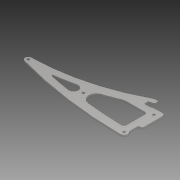
# Autodesk Inventor part: Накладка_4.1.4_3.1_захват(10мм)
Saved by Autodesk Inventor 2016 (Build 200138000, 138)
## iProperties
Created: 2020-03-12
Part Number: Накладка_4.1.4_3.1_захват(10мм)
Material: Поликарбонат, прозрачный
Document SubType Name: Modeling
Designer: Рябов
Density: 1.2 g/cm^3
Appearance: Поликарбонат — прозрачный
Mass: 7.31386 g
Surface Area: 73.6332 cm^2
Volume: 6.09488 cm^3
Author: Рябов
Autodesk Inventor part; units mm, degrees
ref_plane "YZ Plane" through (0, 0, 0) normal (1, 0, 0) x (0, 1, 0)
ref_plane "XZ Plane" through (0, 0, 0) normal (0, 1, 0) x (-1, 0, 0)
ref_plane "XY Plane" through (0, 0, 0) normal (0, 0, 1) x (1, 0, 0)
sketch "Эскиз1" plane through (0, 0, 0) normal (0, 0, 1) x (1, 0, 0)
  circle A0 centre (6.4823, -1.4624) radius 1.65
  circle A1 centre (6.4823, -40.9716) radius 1.65 construction
  arc A2 (-57.7734, 9.189) -> (-62.7021, 3.6942) centre (-59.7433, 5.998) ccw construction
  circle A3 centre (-59.7433, 5.998) radius 1.65 construction
  line L0 (-4.1893, 7.0157) -> (-4.1893, 7.0357) construction
  line L1 (-4.1893, 7.0357) -> (-3.1893, 7.0357) construction
  line L2 (-3.1893, 7.0357) -> (-3.1893, 7.0157) construction
  line L3 (-3.1893, 7.0157) -> (-1.1893, 7.0157) construction
  line L4 (-1.1893, 7.0157) -> (-1.1893, 7.0357) construction
  line L5 (-1.1893, 7.0357) -> (0.8107, 7.0357) construction
  line L6 (0.8107, 7.0357) -> (0.8107, 6.6351) construction
  line L7 (0.8107, 6.6351) -> (-1.1893, 6.6351) construction
  line L8 (-1.1893, 6.6351) -> (-1.1893, 6.6551) construction
  line L9 (-1.1893, 6.6551) -> (-3.1893, 6.6551) construction
  line L10 (-3.1893, 6.6551) -> (-3.1893, 6.6351) construction
  line L11 (-3.1893, 6.6351) -> (-4.1893, 6.6351) construction
  line L12 (-4.1893, 6.6351) -> (-4.1893, 6.6551) construction
  line L13 (-4.1893, 6.6551) -> (-6.1893, 6.6551) construction
  line L14 (-6.1893, 6.6551) -> (-6.1893, 6.6351) construction
  line L15 (-6.1893, 6.6351) -> (-7.1893, 6.6351) construction
  line L16 (-7.1893, 6.6351) -> (-7.1893, 6.6551) construction
  line L17 (-7.1893, 6.6551) -> (-9.1893, 6.6551) construction
  line L18 (-9.1893, 6.6551) -> (-9.1893, 6.6351) construction
  line L19 (-9.1893, 6.6351) -> (-11.1893, 6.6351) construction
  line L20 (-11.1893, 6.6351) -> (-11.1893, 7.0357) construction
  line L21 (-11.1893, 7.0357) -> (-9.1893, 7.0357) construction
  line L22 (-9.1893, 7.0357) -> (-9.1893, 7.0157) construction
  line L23 (-9.1893, 7.0157) -> (-7.1893, 7.0157) construction
  line L24 (-7.1893, 7.0157) -> (-7.1893, 7.0357) construction
  line L25 (-7.1893, 7.0357) -> (-6.1893, 7.0357) construction
  line L26 (-6.1893, 7.0357) -> (-6.1893, 7.0157) construction
  line L27 (-6.1893, 7.0157) -> (-4.1893, 7.0157) construction
  line L28 (-7.6643, 167.4795) -> (-7.6643, 168.8316) construction
  line L29 (-7.6643, 168.8316) -> (-7.1353, 168.8316) construction
  spline S0 degree 3 poles (-7.1353, 168.8316) (-7.0277, 168.8151) (-6.9171, 168.7981) (-6.7021, 168.7651) (-6.5903, 168.748) (-6.4827, 168.7315) knots 0 0 0 0 0.501572 0.501572 1 1 1 1 construction
  line L30 (-6.4827, 168.7315) -> (-3.8958, 168.7315) construction
  spline S1 degree 3 poles (-3.8958, 168.7315) (-3.7882, 168.748) (-3.6765, 168.7651) (-3.4615, 168.7981) (-3.3509, 168.8151) (-3.2433, 168.8316) knots 0 0 0 0 0.498467 0.498467 1 1 1 1 construction
  line L31 (-3.2433, 168.8316) -> (-2.7143, 168.8316) construction
  line L32 (-2.7143, 168.8316) -> (-2.7143, 167.4795) construction
  line L33 (-2.7143, 167.4795) -> (-3.7643, 167.4795) construction
  line L34 (-3.7643, 167.4795) -> (-3.7643, 167.3293) construction
  line L35 (-3.7643, 167.3293) -> (-4.6551, 167.3293) construction
  spline S2 degree 3 poles (-4.6551, 167.3293) (-4.6545, 167.3543) (-4.654, 167.3794) (-4.6529, 167.4294) (-4.6524, 167.4545) (-4.6519, 167.4795) knots 0 0 0 0 0.500007 0.500007 1 1 1 1 construction
  line L36 (-4.6519, 167.4795) -> (-5.7266, 167.4795) construction
  spline S3 degree 3 poles (-5.7266, 167.4795) (-5.7261, 167.4545) (-5.7256, 167.4294) (-5.7245, 167.3794) (-5.724, 167.3543) (-5.7235, 167.3293) knots 0 0 0 0 0.5 0.5 1 1 1 1 construction
  line L37 (-5.7235, 167.3293) -> (-6.6143, 167.3293) construction
  line L38 (-6.6143, 167.3293) -> (-6.6143, 167.4795) construction
  line L39 (-6.6143, 167.4795) -> (-7.6643, 167.4795) construction
  line L40 (0.8107, 166.7784) -> (-11.1893, 166.7784) construction
  line L41 (-11.1893, 166.7784) -> (-11.1893, 167.179) construction
  line L42 (-11.1893, 167.179) -> (-4.3383, 167.179) construction
  spline S4 degree 3 poles (-4.3383, 167.179) (-4.3383, 167.1792) (-4.3383, 167.1794) (-4.3383, 167.1797) (-4.3383, 167.1799) (-4.3383, 167.18) knots 0 0 0 0 0.499986 0.499986 1 1 1 1 construction
  line L43 (-4.3383, 167.18) -> (-4.2964, 167.18) construction
  spline S5 degree 3 poles (-4.2964, 167.18) (-4.2964, 167.1799) (-4.2964, 167.1797) (-4.2963, 167.1794) (-4.2963, 167.1792) (-4.2963, 167.179) knots 0 0 0 0 0.500002 0.500002 1 1 1 1 construction
  line L44 (-4.2963, 167.179) -> (0.8107, 167.179) construction
  line L45 (0.8107, 167.179) -> (0.8107, 166.7784) construction
  line L46 (-11.1893, 6.6251) -> (0.8107, 6.6251) construction
  spline S6 degree 3 poles (0.8107, 6.6251) (0.8107, 6.4396) (0.7674, 6.2212) (0.6255, 5.8786) (0.5021, 5.6936) (0.2685, 5.4598) (0.1339, 5.3598) (-0.0029, 5.2893) knots 0 0 0 0 0.359545 0.359545 0.718791 0.718791 1 1 1 1 construction
  spline S7 degree 3 poles (-0.0029, 5.2893) (-0.2886, 5.142) (-0.5748, 5.01) (-1.5002, 4.6264) (-2.2318, 4.3978) (-3.7268, 4.1001) (-4.4903, 4.0311) (-5.1893, 4.0311) (-5.8883, 4.0311) (-6.6517, 4.1001) (-8.1467, 4.3978) (-8.8784, 4.6264) (-9.8038, 5.01) (-10.0899, 5.142) (-10.3757, 5.2893) knots -0.510232 -0.510232 -0.510232 -0.510232 -0.41941 -0.41941 -0.209705 -0.209705 0 0 0 0.209705 0.209705 0.41941 0.41941 0.510232 0.510232 0.510232 0.510232 construction
  spline S8 degree 3 poles (-10.3757, 5.2893) (-10.5125, 5.3598) (-10.6471, 5.4598) (-10.8806, 5.6936) (-11.0041, 5.8786) (-11.1459, 6.2212) (-11.1893, 6.4396) (-11.1893, 6.6251) knots 0 0 0 0 0.281209 0.281209 0.640455 0.640455 1 1 1 1 construction
  line L47 (0.8107, 167.1891) -> (-11.1893, 167.1891) construction
  spline S9 degree 3 poles (-11.1893, 167.1891) (-11.1893, 167.3746) (-11.1459, 167.5929) (-11.0041, 167.9356) (-10.8806, 168.1206) (-10.6471, 168.3544) (-10.5125, 168.4544) (-10.3757, 168.5249) knots 0 0 0 0 0.359545 0.359545 0.718791 0.718791 1 1 1 1 construction
  spline S10 degree 3 poles (-10.3757, 168.5249) (-10.0899, 168.6722) (-9.8038, 168.8041) (-8.8784, 169.1877) (-8.1467, 169.4164) (-6.6517, 169.714) (-5.8883, 169.7831) (-5.1893, 169.7831) (-4.4903, 169.7831) (-3.7268, 169.714) (-2.2318, 169.4164) (-1.5002, 169.1877) (-0.5748, 168.8041) (-0.2886, 168.6722) (-0.0029, 168.5249) knots -0.510232 -0.510232 -0.510232 -0.510232 -0.41941 -0.41941 -0.209705 -0.209705 0 0 0 0.209705 0.209705 0.41941 0.41941 0.510232 0.510232 0.510232 0.510232 construction
  spline S11 degree 3 poles (-0.0029, 168.5249) (0.1339, 168.4544) (0.2685, 168.3544) (0.5021, 168.1206) (0.6255, 167.9356) (0.7674, 167.5929) (0.8107, 167.3746) (0.8107, 167.1891) knots 0 0 0 0 0.281209 0.281209 0.640455 0.640455 1 1 1 1 construction
  line L48 (0.8107, 7.0357) -> (-11.1893, 7.0357) construction
  line L49 (-11.1893, 7.0357) -> (-11.1893, 9.0391) construction
  line L50 (-11.1893, 9.0391) -> (0.8107, 9.0391) construction
  line L51 (0.8107, 9.0391) -> (0.8107, 7.0357) construction
  line L52 (-11.1893, 166.7784) -> (0.8107, 166.7784) construction
  line L53 (0.8107, 166.7784) -> (0.8107, 164.7751) construction
  line L54 (0.8107, 164.7751) -> (-11.1893, 164.7751) construction
  line L55 (-11.1893, 164.7751) -> (-11.1893, 166.7784) construction
  line L56 (8.8107, -34.9344) -> (8.8107, -18.7776) construction
  arc A4 (10.3107, -17.2776) -> (8.8107, -18.7776) centre (10.3107, -18.7776) ccw construction
  line L57 (10.3107, -17.2776) -> (10.8107, -17.2776) construction
  arc A5 (10.8107, -17.2776) -> (13.3107, -14.7776) centre (10.8107, -14.7776) ccw construction
  arc A6 (8.8107, -34.9344) -> (10.3107, -36.4344) centre (10.3107, -34.9344) ccw construction
  line L58 (10.8107, -36.4344) -> (10.3107, -36.4344) construction
  arc A7 (13.3107, -38.9344) -> (10.8107, -36.4344) centre (10.8107, -38.9344) ccw construction
  circle A8 centre (6.4823, -37.9624) radius 43.5897 construction
  circle A9 centre (6.4823, -37.9624) radius 50.2137 construction
  line L59 (-5.1893, 7.0357) -> (-5.1893, 4.0357) construction
  line L60 (-5.1893, 11.659) -> (-5.1893, 14.7497)
  arc A10 (-5.9418, 10.6901) -> (-10.3994, 9.3285) centre (6.4823, -37.9624) ccw
  circle A11 centre (-129.1063, -19.7124) radius 1.65
  line L61 (-129.1063, -19.7124) -> (-129.1063, -1.4624) construction
  line L62 (-11.1893, 9.0391) -> (-11.1893, 7.6248) construction
  line L63 (-10.1893, 4.0357) -> (-5.3249, 4.0357)
  arc A12 (11.0741, 5.3849) -> (-5.0601, 4.0714) centre (6.4823, -37.9624) ccw
  line L64 (13.3107, 2.8988) -> (13.3107, -14.7776)
  line L65 (0.8107, -46.4344) -> (13.3107, -46.4344) construction
  arc A13 (-130.1181, -23.3233) -> (10.3107, -42.6266) centre (10.3107, 477.8254) ccw
  line L66 (-130.1181, -23.3233) -> (-126.1531, -24.4343) construction
  circle A14 centre (6.4823, -37.9624) radius 52.481 construction
  arc A15 (-10.3994, 9.3285) -> (-11.1893, 7.6248) centre (-10.4822, 8.3319) ccw
  line L67 (-11.1893, 9.0391) -> (-10.4822, 8.3319) construction
  arc A16 (-11.1893, 5.0357) -> (-10.1893, 4.0357) centre (-10.1893, 5.0357) ccw
  arc A17 (-5.3249, 4.0357) -> (-5.0601, 4.0714) centre (-5.3249, 5.0357) ccw
  arc A18 (13.3107, 2.8988) -> (11.0741, 5.3849) centre (10.8107, 2.8988) ccw
  arc A19 (-5.1893, 14.7497) -> (-6.1893, 15.7497) centre (-6.1893, 14.7497) ccw
  arc A20 (-5.9418, 10.6901) -> (-5.1893, 11.659) centre (-6.1893, 11.659) ccw
  line L68 (0.8107, -29.4726) -> (0.8107, -6.9643)
  line L69 (-26.5073, -3.9643) -> (-2.1893, -3.9643)
  line L70 (0.8107, 32.412) -> (0.8107, -57.5372) construction
  arc A21 (-85.3429, -21.6168) -> (-46.8702, -11.5877) centre (-133.6856, 242.6386) ccw construction
  arc A22 (-90.6769, -22.5372) -> (-44.87, -29.6352) centre (10.3107, 477.8254) ccw construction
  arc A23 (0.8107, -6.9643) -> (-2.1893, -3.9643) centre (-2.1893, -6.9643) ccw
  arc A24 (-26.5073, -3.9643) -> (-27.6909, -4.2076) centre (-26.5073, -6.9643) ccw
  arc A25 (-46.8702, -11.5877) -> (-44.87, -29.6352) centre (-43.8646, -20.3892) ccw
  arc A26 (-2.2632, -32.4717) -> (0.8107, -29.4726) centre (-2.1893, -29.4726) ccw
  line L71 (10.8107, -34.356) -> (10.3107, -34.356)
  line L72 (8.8107, -32.856) -> (8.8107, -20.856)
  line L73 (10.3107, -19.356) -> (10.8107, -19.356)
  line L74 (13.3107, -16.856) -> (13.3107, -14.7776)
  arc A27 (10.8107, -19.356) -> (13.3107, -16.856) centre (10.8107, -16.856) ccw
  arc A28 (13.3107, -36.856) -> (10.8107, -34.356) centre (10.8107, -36.856) ccw
  arc A29 (10.3107, -19.356) -> (8.8107, -20.856) centre (10.3107, -20.856) ccw
  arc A30 (8.8107, -32.856) -> (10.3107, -34.356) centre (10.3107, -32.856) ccw
  circle A31 centre (6.4823, -37.9624) radius 1.65
  arc A32 (10.3107, -42.6266) -> (13.3107, -39.6266) centre (10.3107, -39.6266) ccw
  line L75 (13.3107, -36.856) -> (13.3107, -39.6266)
  line L76 (12.3341, -42.6266) -> (-36.8572, -42.6266) construction
  arc A33 (-10.3994, 9.3285) -> (-11.1893, 9.0391) centre (6.4823, -37.9624) ccw construction
  line L77 (-11.1893, 7.6248) -> (-11.1893, 5.0357)
  arc A34 (-129.1717, -15.9629) -> (-12.3839, 14.2069) centre (-133.6856, 242.6386) ccw
  arc A35 (-129.1717, -15.9629) -> (-130.1181, -23.3233) centre (-129.1063, -19.7124) ccw
  arc A36 (-5.1667, 16.0085) -> (-12.0803, 14.0375) centre (6.4823, -37.9624) ccw construction
  arc A37 (-6.1893, 15.7497) -> (-12.3839, 14.2069) centre (-6.1893, 2.5413) ccw
  line L78 (-6.1893, 15.7497) -> (-16.5229, 15.7497) construction
  line L79 (6.4823, -1.4624) -> (6.4823, -37.9624) construction
  line L80 (-129.1717, -15.9629) -> (-45.0288, -14.4942) construction
  line L81 (13.3107, -168.3488) -> (-132.8563, -168.3488) construction
  line L82 (-132.8563, -168.3488) -> (-132.8563, -116.6071) construction
  circle A38 centre (-59.7728, -21.5513) radius 1.65
  circle A39 centre (-59.7728, -21.5513) radius 6.65 construction
  line L83 (-59.7728, -5.2162) -> (-59.7728, -37.8863) construction
  arc A40 (-46.8702, -11.5877) -> (-27.6909, -4.2076) centre (-133.6856, 242.6386) ccw
  arc A41 (-44.87, -29.6352) -> (-2.2632, -32.4717) centre (10.3107, 477.8254) ccw
  arc A42 (-99.3569, -21.279) -> (-99.4418, -23.2475) centre (-99.2279, -22.2707) ccw
  arc A43 (-73.287, -28.2686) -> (-73.6579, -16.6444) centre (-72.3209, -22.4197) ccw
  arc A44 (-99.3569, -21.279) -> (-73.6579, -16.6444) centre (-133.6856, 242.6386) ccw
  arc A45 (-99.4418, -23.2475) -> (-73.287, -28.2686) centre (10.3107, 477.8254) ccw
  point P0 (0, 0)
  point P1 (-5.1893, 10.8761)
  point P2 (-5.1893, 16.0036)
  point P3 (-5.1893, 9.0391)
  point P4 (13.3107, 5.0892)
  point P5 (13.3107, -46.4344)
  point P6 (0.8107, -42.5398)
  point P7 (-35.4501, -6.404)
  point P8 (-71.9591, -10.0794)
  point P9 (-5.1893, 13.2043)
  point P10 (-8.669, 12.284)
  point P11 (0.8107, -32.5381)
  point P12 (0.8107, -3.9643)
  point P13 (-27.1259, -3.9643)
  point P14 (0.8107, -32.5381)
  point P15 (8.8107, -34.356)
  point P16 (8.8107, -19.356)
  point P17 (13.3107, -19.356)
  point P18 (8.8107, -26.856)
  point P19 (6.4823, -19.7124)
  point P20 (-59.7728, -168.3488)
  dimension "d0" = 3
  dimension "d12" = 45
  dimension "d13" = 2
  dimension "d14" = 1
  dimension "d17" = 1
  dimension "d23" = 10
  dimension "d25" = 8
  dimension "d26" = 3
  dimension "d27" = 15
  dimension "d31" = 3
  dimension "d33" = 36.5
  dimension "d36" = 3
  dimension "d39" = 7.5
  dimension "d41" = 10
  dimension "d42" = 5
  dimension "d48" = 5
  dimension "d50" = 91
  dimension "d51" = 69.363
  dimension "d61" = 3.3
  dimension "d64" = 5
  dimension "d68" = 1
  dimension "d69" = 7.5
  dimension "d70" = 7.5
  constraints: 159 end point, 82 point on circle, 46 tangent, 38 centre point, 35 horizontal, 33 vertical, 24 point on line, 11 equal radius, 8 midpoint, 7 coincident, 6 perpendicular, 3 concentric, 3 vertical alignment, 1 collinear, 1 horizontal alignment, 98 other
  measures "d0" distance of L59.start L59.end
  measures "d12" angle of L62 L67
  measures "d13" diameter of A15
  measures "d14" radius of A16
  measures "d17" radius of A19
  measures "d23" radial gap between concentric circles of A13 A22
  measures "d25" distance between parallel lines of L69 L63
  measures "d26" radius of A23
  measures "d27" distance between parallel lines of L71 L73
  measures "d31" radius of A32
  measures "d33" distance of A8.centre L79.start
  measures "d39" diameter of A35
  measures "d41" radial gap between concentric circles of A34 A21
  measures "d42" radial gap between concentric circles of A10 A36
  measures "d50" angle of L61 L80
  measures "d51" distance from line of L61 A2.centre
  measures "d61" diameter of A38
  measures "d68" radius of A42
  measures "d69" radial gap between concentric circles of A13 A45
  measures "d70" radial gap between concentric circles of A34 A44
extrude "Выдавливание1" add sketch "Эскиз1" against normal blind 2
fillet "Сопряжение1" radius 1 2 edges at (-11.1893, 7.6248, -1) (-10.3994, 9.3285, -1)
move faces "Перенос1" translate (0, -3.5, 0) faces at (10.4774, -19.356, -0.6667)
delete faces "Удаление грани1" heal yes whole lump no faces at (9.4658, -34.0953, -1.3333) (10.6441, -34.356, -0.6667) (12.8763, -35.4477, -1.3333)
sketch "Эскиз3" plane through (-10.1893, 4.0357, 0) normal (0, 0, 1) x (1, 0, 0)
  line L0 (19, -46.6601) -> (19, -28.3917) projected
  arc A0 (20.5, -26.8917) -> (19, -28.3917) centre (20.5, -28.3917) ccw projected
  line L1 (20.5, -26.8917) -> (21, -26.8917) projected
  arc A1 (21, -26.8917) -> (23.5, -24.3917) centre (21, -24.3917) ccw projected
  line L2 (23.5, -24.3917) -> (23.5, -1.137) projected
  arc A2 (23.5, -1.137) -> (21.2634, 1.3491) centre (21, -1.137) ccw projected
  arc A3 (21.2634, 1.3491) -> (5.1292, 0.0357) centre (16.6716, -41.9981) ccw projected
  arc A4 (4.8644, 0) -> (5.1292, 0.0357) centre (4.8644, 1) ccw projected
  line L3 (4.8644, 0) -> (0, 0) projected
  arc A5 (-1, 1) -> (0, 0) centre (0, 1) ccw projected
  line L4 (-1, 1) -> (-1, 3.2542) projected
  arc A6 (-1, 3.2542) -> (-1.1464, 3.7752) centre (-2, 3.2542) ccw projected
  arc A7 (-0.3353, 5.2953) -> (-1.1464, 3.7752) centre (-0.2929, 4.2962) ccw projected
  arc A8 (-0.3353, 5.2953) -> (-0.0448, 5.3514) centre (-0.3777, 6.2944) ccw projected
  arc A9 (4.2474, 6.6543) -> (-0.0448, 5.3514) centre (16.6716, -41.9981) ccw projected
  arc A10 (4.2474, 6.6543) -> (5, 7.6232) centre (4, 7.6232) ccw projected
  line L5 (5, 7.6232) -> (5, 10.7139) projected
  arc A11 (5, 10.7139) -> (4, 11.7139) centre (4, 10.7139) ccw projected
  arc A12 (4, 11.7139) -> (-2.1947, 10.1712) centre (4, -1.4944) ccw projected
  arc A13 (-118.9824, -19.9987) -> (-2.1947, 10.1712) centre (-123.4964, 238.6029) ccw projected
  arc A14 (-118.9824, -19.9987) -> (-119.9288, -27.359) centre (-118.917, -23.7481) ccw projected
  arc A15 (-119.9288, -27.359) -> (19, -46.6601) centre (20.5, 473.7897) ccw projected
  arc A16 (-16.318, -8) -> (-17.5017, -8.2434) centre (-16.318, -11) ccw projected
  line L6 (-16.318, -8) -> (8, -8) projected
  arc A17 (11, -11) -> (8, -8) centre (8, -11) ccw projected
  line L7 (11, -11) -> (11, -33.5083) projected
  arc A18 (7.9261, -36.5074) -> (11, -33.5083) centre (8, -33.5083) ccw projected
  arc A19 (-34.6808, -33.671) -> (7.9261, -36.5074) centre (20.5, 473.7897) ccw projected
  arc A20 (-36.681, -15.6235) -> (-34.6808, -33.671) centre (-33.6754, -24.425) ccw projected
  arc A21 (-36.681, -15.6235) -> (-17.5017, -8.2434) centre (-123.4964, 238.6029) ccw projected
  arc A22 (-89.2526, -27.2833) -> (-63.0977, -32.3043) centre (20.5, 473.7897) ccw projected
  arc A23 (-89.1676, -25.3148) -> (-89.2526, -27.2833) centre (-89.0386, -26.3064) ccw projected
  arc A24 (-89.1676, -25.3148) -> (-63.4687, -20.6801) centre (-123.4964, 238.6029) ccw projected
  arc A25 (-63.0977, -32.3043) -> (-63.4687, -20.6801) centre (-62.1316, -26.4555) ccw projected
  circle A26 centre (-49.5835, -25.587) radius 1.65 projected
  circle A27 centre (16.6716, -41.9981) radius 1.65 projected
  circle A28 centre (-118.917, -23.7481) radius 1.65 projected
  circle A29 centre (16.6716, -5.4981) radius 1.65 projected
  arc A30 (16.6371, -46.648) -> (19, -46.0231) centre (16.6716, -41.9981) ccw
  arc A31 (-119.9288, -27.359) -> (19, -46.6601) centre (20.5, 473.7897) ccw projected
  arc A32 (19, -46.0231) -> (19, -37.9731) centre (16.6716, -41.9981) ccw
  point P0 (10.1893, -4.0357)
  constraints: 5 point on circle, 2 centre point, 2 point on line, 1 coincident, 1 tangent
extrude "Выдавливание3" cut sketch "Эскиз3" against normal blind 10 contours A15 A30 L0
extrude "Выдавливание4" add sketch "Эскиз3" against normal up to surface (2 mm away) contours L0 A32
fillet "Сопряжение2" radius 3 1 edges at (8.8107, -33.9373, -1)
delete faces "Удаление грани2" heal yes whole lump no faces at (-68.5025, -26.9543, -1.3333) (-99.517, -23.228, -1.3333) (-96.5491, -23.8724, -0.6667) (-96.4805, -20.8889, -1.3333)
delete faces "Удаление грани3" heal yes whole lump no faces at (-2.0353, -32.4686, -0.6667) (0.8107, -21.9698, -0.6667) (-21.2282, -31.6513, -1.3333) (-1.9651, -3.9726, -1.3333) (-10.2953, -3.9643, -0.6667) (-27.1775, -4.0401, -1.3333) (-38.2766, -8.489, -1.3333) (-45.6235, -29.5219, -1.3333)
sketch "Эскиз9" plane through (-10.1893, 4.0357, 0) normal (0, 0, 1) x (1, 0, 0)
  circle A0 centre (16.6716, -5.4981) radius 1.65 construction
  circle A1 centre (-118.917, -23.7481) radius 1.65 construction
  circle A2 centre (16.6716, -41.9981) radius 1.65 construction
  circle A3 centre (-49.5835, -25.587) radius 1.65 construction
  arc A4 (16.6371, -46.648) -> (19.9104, -38.6616) centre (16.6716, -41.9981) ccw construction
  arc A5 (19, -36.509) -> (19.9104, -38.6616) centre (22, -36.509) ccw construction
  line L0 (19, -36.509) -> (19, -28.3917) construction
  arc A6 (20.5, -26.8917) -> (19, -28.3917) centre (20.5, -28.3917) ccw construction
  line L1 (20.5, -26.8917) -> (21, -26.8917) construction
  arc A7 (21, -26.8917) -> (23.5, -24.3917) centre (21, -24.3917) ccw construction
  line L2 (23.5, -24.3917) -> (23.5, -1.137) construction
  arc A8 (23.5, -1.137) -> (21.2634, 1.3491) centre (21, -1.137) ccw construction
  arc A9 (21.2634, 1.3491) -> (5.1292, 0.0357) centre (16.6716, -41.9981) ccw construction
  arc A10 (4.8644, 0) -> (5.1292, 0.0357) centre (4.8644, 1) ccw construction
  line L3 (4.8644, 0) -> (0, 0) construction
  arc A11 (-1, 1) -> (0, 0) centre (0, 1) ccw construction
  line L4 (-1, 1) -> (-1, 3.2542) construction
  arc A12 (-1, 3.2542) -> (-1.1464, 3.7752) centre (-2, 3.2542) ccw construction
  arc A13 (-0.3353, 5.2953) -> (-1.1464, 3.7752) centre (-0.2929, 4.2962) ccw construction
  arc A14 (-0.3353, 5.2953) -> (-0.0448, 5.3514) centre (-0.3777, 6.2944) ccw construction
  arc A15 (4.2474, 6.6543) -> (-0.0448, 5.3514) centre (16.6716, -41.9981) ccw construction
  arc A16 (4.2474, 6.6543) -> (5, 7.6232) centre (4, 7.6232) ccw construction
  line L5 (5, 7.6232) -> (5, 10.7139) construction
  arc A17 (5, 10.7139) -> (4, 11.7139) centre (4, 10.7139) ccw construction
  arc A18 (4, 11.7139) -> (-2.1947, 10.1712) centre (4, -1.4944) ccw construction
  arc A19 (-118.9824, -19.9987) -> (-2.1947, 10.1712) centre (-123.4964, 238.6029) ccw construction
  arc A20 (-118.9824, -19.9987) -> (-119.9288, -27.359) centre (-118.917, -23.7481) ccw construction
  arc A21 (-119.9288, -27.359) -> (16.6371, -46.648) centre (20.5, 473.7897) ccw construction
  line L6 (11, -33.5083) -> (11, -11)
  line L7 (8, -8) -> (-13.8783, -8)
  arc A22 (-37.8231, -16.0107) -> (-19.6753, -9.1655) centre (-123.4964, 238.6029) ccw
  arc A23 (-35.9431, -33.5321) -> (7.9261, -36.5074) centre (20.5, 473.7897) ccw
  arc A24 (-118.9824, -19.9987) -> (-2.1947, 10.1712) centre (-123.4964, 238.6029) ccw construction
  line L8 (-16.9366, -8) -> (-20.9033, 1.1796) construction
  line L9 (-20.9033, 1.1796) -> (-20.0703, 1.5396) construction
  line L10 (11, -36.5739) -> (10.8139, -46.5722) construction
  line L11 (10.8139, -46.5722) -> (3.4115, -46.4344) construction
  arc A25 (-119.9288, -27.359) -> (16.6371, -46.648) centre (20.5, 473.7897) ccw construction
  arc A26 (-37.8231, -16.0107) -> (-35.9431, -33.5321) centre (-34.9452, -24.5635) ccw
  circle A27 centre (-49.5835, -25.587) radius 5.65 construction
  arc A28 (-87.0352, -25.0286) -> (-62.3359, -20.4153) centre (-123.4964, 238.6029) ccw
  arc A29 (-87.1082, -26.9969) -> (-61.9377, -31.7504) centre (20.5, 473.7897) ccw
  arc A30 (-61.9377, -31.7504) -> (-62.3359, -20.4153) centre (-61.007, -26.0431) ccw
  circle A31 centre (-118.917, -23.7481) radius 1.65 projected
  arc A32 (-118.917, -23.7481) -> (-34.9452, -24.5635) centre (-72.7119, 410.3709) ccw construction
  arc A33 (-87.0352, -25.0286) -> (-87.1082, -26.9969) centre (-86.8982, -26.0192) ccw
  arc A34 (11, -11) -> (8, -8) centre (8, -11) ccw
  arc A35 (7.9261, -36.5074) -> (11, -33.5083) centre (8, -33.5083) ccw
  arc A36 (-13.8783, -8) -> (-19.6753, -9.1655) centre (-13.8783, -23) ccw
  point P0 (10.1893, -4.0357)
  dimension "d110" = 8
  dimension "d111" = 8
  dimension "d112" = 10
  dimension "d114" = 4
  dimension "d115" = 1
  dimension "d116" = 7.5
  dimension "d117" = 3
  dimension "d118" = 15
  constraints: 28 point on circle, 16 tangent, 12 centre point, 12 end point, 4 concentric, 2 perpendicular, 2 point on line, 1 coincident, 1 equal length, 1 equal radius, 1 horizontal, 1 vertical
  measures "d110" distance between parallel lines of L0 L6
  measures "d111" distance between parallel lines of L7 L3
  measures "d112" radial gap between concentric circles of A19 A22
  measures "d114" radial gap between concentric circles of A3 A27
  measures "d115" radius of A33
  measures "d116" radial gap between concentric circles of A19 A28
  measures "d117" radius of A34
  measures "d118" radius of A36
extrude "Выдавливание9" cut sketch "Эскиз9" against normal blind 10 contours A35 A23 A26 A22 A36 L7 A34 L6 | A28 A30 A29 A33
